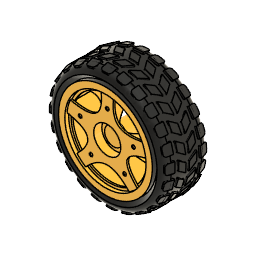
Rubber wheel (Autodesk Fusion 360 design; units mm, degrees)
part number: 2025-09-30-12-13-26-150
Autodesk Fusion 360 part; units mm, degrees
sketch "Sketch3" plane through (0, 0, 0) normal (0, 1, 0) x (1, 0, 0)
  circle A0 centre (0, 0) radius 26
  circle A1 centre (0, 0) radius 22.5
  dimension "d5" = 52
  dimension "d6" = 45
  constraint coincident A0.centre A1.centre
  measures "d5" diameter of A0
  measures "d6" diameter of A1
extrude "Extrude2" add sketch "Sketch3" along normal blind 25 makes body 1
sketch "Sketch4" plane through (0, 0, 0) normal (0, 1, 0) x (1, 0, 0)
  circle A0 centre (0, 0) radius 22.39
  dimension "d9" = 44.78
  constraint coincident A0.centre origin
  measures "d9" diameter of A0
extrude "Extrude3" add sketch "Sketch4" along normal blind 25 separate body makes body 2
sketch "Sketch5" plane through (0, 25, 0) normal (0, 1, 0) x (-1, 0, 0)
  circle A0 centre (0, 0) radius 22.39
  circle A1 centre (0, 0) radius 21
  dimension "d12" = 42
  constraint concentric A0 A1
  measures "d12" diameter of A1
extrude "Extrude4" cut sketch "Sketch5" against normal blind 20 contours A1 bodies 2
sketch "Sketch6" plane through (0, 0, 0) normal (0, 1, 0) x (1, 0, 0)
  circle A0 centre (0, 0) radius 21
  dimension "d15" = 42
  constraint coincident A0.centre origin
  measures "d15" diameter of A0
extrude "Extrude5" cut sketch "Sketch6" along normal blind 4 bodies 2
extrude "Extrude6" cut 1 faces at (-5.9246, 4, -2.0633) along direction (0, 1, 0) blind 1 on bodies 2 bodies 2
extrude "Extrude7" cut 1 faces at (21.7651, 25, 2.1556) along direction (0, -1, 0) blind 20 on bodies 2 bodies 2
extrude "Extrude8" cut 1 faces at (21.8433, 0, 1.1124) along direction (0, 1, 0) blind 4 on bodies 2 bodies 2
sketch "Sketch7" plane through (0, 0, 0) normal (0, 1, 0) x (1, 0, 0)
  circle A0 centre (0, 0) radius 9
  dimension "d24" = 18
  constraint coincident A0.centre origin
  measures "d24" diameter of A0
extrude "Extrude9" add sketch "Sketch7" along normal blind 25 separate body makes body 3
sketch "Sketch8" plane through (0, 0, 0) normal (0, 1, 0) x (1, 0, 0)
  circle A0 centre (0, 0) radius 7.5
  dimension "d27" = 15
  constraint coincident A0.centre origin
  measures "d27" diameter of A0
extrude "Extrude10" cut sketch "Sketch8" along normal blind 4 bodies 3
sketch "Sketch9" plane through (0, 25, 0) normal (0, 1, 0) x (-1, 0, 0)
  circle A0 centre (0, 0) radius 9
  circle A1 centre (0, 0) radius 5
  dimension "d30" = 10
  constraint coincident A0.centre A1.centre
  measures "d30" diameter of A1
extrude "Extrude11" cut sketch "Sketch9" against normal blind 20 bodies 3
sketch "Sketch10" plane through (0, 25, 0) normal (0, 1, 0) x (-1, 0, 0)
  circle A0 centre (0, 0) radius 5
  circle A1 centre (0, 0) radius 3
  dimension "d33" = 6
  constraint coincident A0.centre A1.centre
  measures "d33" diameter of A1
extrude "Extrude12" cut sketch "Sketch10" against normal blind 20 contours A1 bodies 3
sketch "Sketch11" plane through (0, 0, 0) normal (0, 1, 0) x (1, 0, 0)
  circle A0 centre (0, 0) radius 5
  dimension "d36" = 10
  constraint coincident A0.centre origin
  measures "d36" diameter of A0
extrude "Extrude13" add sketch "Sketch11" along normal blind 4 bodies 3
extrude "Extrude14" cut 1 faces at (1.3101, 0, 1.9935) along direction (0, 1, 0) blind 3 on bodies 3 bodies 3
sketch "Sketch12" plane through (0, 0, 0) normal (0, 1, 0) x (1, 0, 0)
  circle A0 centre (-4, -5) radius 0.5
  circle A1 centre (4, -5) radius 0.5
  circle A2 centre (-4, 5) radius 0.5
  circle A3 centre (4, 5) radius 0.5
  dimension "d41" = 1
  dimension "d42" = 1
  dimension "d43" = 1
  dimension "d44" = 1
  measures "d41" diameter of A0
  measures "d42" diameter of A1
  measures "d43" diameter of A2
  measures "d44" diameter of A3
extrude "Extrude15" add sketch "Sketch12" along normal blind 4 bodies 3
extrude "Extrude16" cut 4 faces at (-3.8778, 0, 5.1472) (4.1222, 0, 4.8866) (4.1222, 0, -5.1134) (-3.8778, 0, -4.8528) along direction (0, 1, 0) blind 3.5 on bodies 3 bodies 3
extrude "Extrude17" cut 1 faces at (1.3101, 3, 1.9935) along direction (0, 1, 0) blind 0.5 on bodies 3 bodies 3
extrude "Extrude18" cut 1 faces at (-2.7054, 4, 5.6176) along direction (0, 1, 0) blind 0.5 on bodies 3 bodies 3
extrude "Extrude19" cut 1 faces at (4.1222, 3.5, 4.8866) along direction (0, 1, 0) blind 0.5 on bodies 3 bodies 3
extrude "Extrude20" cut 3 faces at (-3.8778, 3.5, 5.1472) (-3.8778, 3.5, -4.8528) (4.1222, 3.5, -5.1134) along direction (0, 1, 0) blind 0.5 on bodies 3 bodies 3
extrude "Extrude21" cut 1 faces at (8.4386, 0, 0.8197) along direction (0, 1, 0) blind 0.5 on bodies 3 bodies 3
extrude "Extrude22" add 1 faces at (21.8433, 4, 1.1124) along direction (0, -1, 0) blind 0.5 on bodies 2 bodies 2
extrude "Extrude23" add 1 faces at (21.8433, 3.5, 1.1124) along direction (0, -1, 0) blind 1.5 on bodies 2 bodies 2
extrude "Extrude24" add 1 faces at (7.6145, 5, 0.6955) along direction (0, 1, 0) blind 1 on bodies 3 bodies 3
extrude "Extrude25" cut 1 faces at (1.3101, 3.5, 1.9935) along direction (0, 1, 0) blind 0.5 on bodies 3 bodies 3
extrude "Extrude26" cut 1 faces at (-2.7054, 4.5, 5.6176) along direction (0, 1, 0) blind 0.5 on bodies 3 bodies 3
extrude "Extrude27" cut 4 faces at (4.1222, 4, 4.8866) (-3.8778, 4, 5.1472) (-3.8778, 4, -4.8528) (4.1222, 4, -5.1134) along direction (0, 1, 0) blind 0.5 on bodies 3 bodies 3
extrude "Extrude28" cut 1 faces at (8.4386, 0.5, 0.8197) along direction (0, 1, 0) blind 0.5 on bodies 3 bodies 3
extrude "Extrude29" cut 1 faces at (1.3101, 4, 1.9935) along direction (0, 1, 0) blind 0.5 on bodies 3 bodies 3
extrude "Extrude30" cut 1 faces at (-2.7054, 5, 5.6176) along direction (0, 1, 0) blind 0.5 on bodies 3 bodies 3
extrude "Extrude31" cut 4 faces at (4.1222, 4.5, 4.8866) (-3.8778, 4.5, 5.1472) (-3.8778, 4.5, -4.8528) (4.1222, 4.5, -5.1134) along direction (0, 1, 0) blind 0.5 on bodies 3 bodies 3
extrude "Extrude32" cut 1 faces at (8.4386, 1, 0.8197) along direction (0, 1, 0) blind 0.5 on bodies 3 bodies 3
extrude "Extrude33" cut 1 faces at (21.7651, 5, 2.1556) along direction (0, -1, 0) blind 2 on bodies 2 bodies 2
sketch "Sketch14" plane through (0, 2, 0) normal (0, -1, 0) x (1, 0, 0)
  circle A0 centre (0, 0) radius 21
  circle A1 centre (0, 0) radius 22.39
  spline S0 degree 5 poles (-3.4973, 22.1152) (-3.4006, 21.4068) (-3.2459, 20.0296) (-3.1304, 18.0828) (-3.213, 15.729) (-3.7369, 13.2166) (-4.7167, 11.17) (-6.186, 9.6237) (-8.1564, 8.5893) (-10.6008, 8.0394) (-13.4805, 7.9342) (-16.1022, 8.1751) (-18.2359, 8.5267) (-19.7314, 8.8358) (-20.4975, 9.0091) knots 0 0 0 0 0 0 0.1 0.2 0.3 0.4 0.5 0.6 0.7 0.8 0.9 1 1 1 1 1 1
  spline S1 degree 5 poles (3.5817, 22.1017) (3.4802, 21.3937) (3.3163, 20.0174) (3.1876, 18.0719) (3.2545, 15.7198) (3.7619, 13.2094) (4.7285, 11.1648) (6.1881, 9.6202) (8.1522, 8.5873) (10.5935, 8.0385) (13.4729, 7.934) (16.0965, 8.1752) (18.2326, 8.5268) (19.7303, 8.8359) (20.4975, 9.0091) knots 0 0 0 0 0 0 0.1 0.2 0.3 0.4 0.5 0.6 0.7 0.8 0.9 1 1 1 1 1 1
  spline S2 degree 5 poles (-22.2999, 2.0065) (-21.5457, 1.858) (-20.0933, 1.5448) (-18.0826, 1.0258) (-15.7431, 0.2342) (-13.4268, -0.9327) (-11.7736, -2.2931) (-10.839, -3.8632) (-10.6558, -5.6526) (-11.1973, -7.6534) (-12.41, -9.8502) (-13.8739, -11.7516) (-15.2319, -13.2536) (-16.2509, -14.2882) (-16.7889, -14.8137) knots 0 0 0 0 0 0 0.1 0.2 0.3 0.4 0.5 0.6 0.7 0.8 0.9 1 1 1 1 1 1
  spline S3 degree 5 poles (-11.9561, -18.9305) (-11.4797, -18.4067) (-10.5263, -17.4047) (-9.0948, -16.0384) (-7.1832, -14.4945) (-4.7882, -13.0593) (-2.3875, -12.1628) (0.0196, -11.8488) (2.4332, -12.1407) (4.8531, -13.0142) (7.2788, -14.4252) (9.2236, -15.9486) (10.6845, -17.2991) (11.6593, -18.2903) (12.147, -18.8086) knots 0 0 0 0 0 0 0.1 0.2 0.3 0.4 0.5 0.6 0.7 0.8 0.9 1 1 1 1 1 1
  spline S4 degree 5 poles (22.2946, 2.0646) (21.5424, 1.9146) (20.0936, 1.5981) (18.0874, 1.0738) (15.7518, 0.2739) (13.4367, -0.9054) (11.7808, -2.2803) (10.8389, -3.8673) (10.6436, -5.676) (11.168, -7.6984) (12.3591, -9.9187) (13.8022, -11.8404) (15.1427, -13.3585) (16.1494, -14.404) (16.6809, -14.9352) knots 0 0 0 0 0 0 0.1 0.2 0.3 0.4 0.5 0.6 0.7 0.8 0.9 1 1 1 1 1 1
  point P0 (-6, 10)
  point P1 (6, 10)
  point P2 (-11, -4)
  point P3 (0, -12)
  point P4 (11, -4)
  constraint coincident A1 S0.start
  constraint coincident A1 S0.end
  constraint coincident A1 S1.start
  constraint coincident A1 S1.end
  constraint coincident A1 S2.start
  constraint coincident A1 S2.end
  constraint coincident A1 S3.start
  constraint coincident A1 S3.end
  constraint coincident A1 S4.start
  constraint coincident A1 S4.end
extrude "Extrude34" add sketch "Sketch14" along normal blind 0.01 contours A0 S0 S1 S2 S3 S4 | A0 A1 S1 S4 | A0 A1 S3 S4 | A0 A1 S0 S1 | A0 A1 S2 S3 | A0 A1 S0 S2 bodies 2 3
extrude "Extrude35" add 1 faces at (8.4386, 1.5, 0.8197) along direction (0, -1, 0) blind 0.5 on bodies 2 bodies 2
extrude "Extrude36" add 1 faces at (-12.1299, 1.99, 3.4531) along direction (0, -1, 0) blind 0.95 on bodies 2 bodies 2
extrude "Extrude37" add 1 faces at (-12.1299, 1.04, 3.4531) along direction (0, -1, 0) blind 0.04 on bodies 2 bodies 2
extrude "Extrude38" cut 1 faces at (1.9158, 1.99, 2.8099) along direction (0, 1, 0) blind 2 on bodies 2 bodies 2
fillet "Fillet1" radius 3 1 edges at (-8.3909, 6, 3.2545) on bodies 2
sketch "Sketch15" plane through (0, 2, 0) normal (0, 1, 0) x (-1, 0, 0)
  circle A0 centre (0, 0) radius 9
  arc A1 (-19.1063, 8.7148) -> (-20.9251, 1.7721) centre (0, 0) ccw
  spline S0 degree 5 poles (-20.9251, 1.7721) (-20.4807, 1.6705) (-19.3542, 1.3982) (-17.6543, 0.9227) (-15.5784, 0.1856) (-13.4367, -0.9054) (-11.7808, -2.2803) (-10.8389, -3.8673) (-10.6436, -5.676) (-11.168, -7.6984) (-12.2684, -9.7495) (-13.5318, -11.4758) (-14.6447, -12.784) (-15.4072, -13.6149) (-15.7096, -13.9358) knots 0.037451 0.037451 0.037451 0.037451 0.037451 0.037451 0.1 0.2 0.3 0.4 0.5 0.6 0.7 0.8 0.9 0.961913 0.961913 0.961913 0.961913 0.961913 0.961913
  arc A2 (-15.7096, -13.9358) -> (-11.1555, -17.792) centre (0, 0) ccw
  spline S1 degree 5 poles (10.9829, -17.899) (10.7008, -17.6112) (9.9416, -16.8584) (8.7045, -15.7273) (6.9876, -14.3773) (4.7882, -13.0593) (2.3875, -12.1628) (-0.0196, -11.8488) (-2.4332, -12.1407) (-4.8531, -13.0142) (-7.0814, -14.3104) (-8.8281, -15.6429) (-10.0903, -16.7612) (-10.8664, -17.5065) (-11.1555, -17.792) knots 0.040836 0.040836 0.040836 0.040836 0.040836 0.040836 0.1 0.2 0.3 0.4 0.5 0.6 0.7 0.8 0.9 0.959321 0.959321 0.959321 0.959321 0.959321 0.959321
  arc A3 (10.9829, -17.899) -> (15.8065, -13.8258) centre (0, 0) ccw
  spline S2 degree 5 poles (20.9296, 1.7176) (20.4835, 1.617) (19.3537, 1.3473) (17.6496, 0.8766) (15.57, 0.147) (13.4268, -0.9327) (11.7736, -2.2931) (10.839, -3.8632) (10.6558, -5.6526) (11.1973, -7.6534) (12.3177, -9.683) (13.5998, -11.3912) (14.7277, -12.6858) (15.5001, -13.5081) (15.8065, -13.8258) knots 0.037374 0.037374 0.037374 0.037374 0.037374 0.037374 0.1 0.2 0.3 0.4 0.5 0.6 0.7 0.8 0.9 0.961948 0.961948 0.961948 0.961948 0.961948 0.961948
  arc A4 (20.9296, 1.7176) -> (19.1065, 8.7144) centre (0, 0) ccw
  spline S3 degree 5 poles (3.3353, 20.7335) (3.2958, 20.3268) (3.2093, 19.2625) (3.1502, 17.6167) (3.2548, 15.5285) (3.7369, 13.2166) (4.7167, 11.17) (6.186, 9.6237) (8.1564, 8.5893) (10.6008, 8.0394) (13.2675, 7.942) (15.6203, 8.1333) (17.4548, 8.4045) (18.6407, 8.6226) (19.1065, 8.7144) knots 0.039901 0.039901 0.039901 0.039901 0.039901 0.039901 0.1 0.2 0.3 0.4 0.5 0.6 0.7 0.8 0.9 0.963032 0.963032 0.963032 0.963032 0.963032 0.963032
  arc A5 (3.3353, 20.7335) -> (-3.4104, 20.7212) centre (0, 0) ccw
  spline S4 degree 5 poles (-3.4104, 20.7212) (-3.3681, 20.3147) (-3.2745, 19.251) (-3.2043, 17.6062) (-3.295, 15.5195) (-3.7619, 13.2094) (-4.7285, 11.1648) (-6.1881, 9.6202) (-8.1522, 8.5873) (-10.5935, 8.0385) (-13.2603, 7.9418) (-15.6149, 8.1334) (-17.4516, 8.4048) (-18.6395, 8.623) (-19.1063, 8.7148) knots 0.039888 0.039888 0.039888 0.039888 0.039888 0.039888 0.1 0.2 0.3 0.4 0.5 0.6 0.7 0.8 0.9 0.963081 0.963081 0.963081 0.963081 0.963081 0.963081
  line L0 (0.4907, 5.8974) -> (-0.5093, 5.8974)
  line L1 (-0.5093, 5.8974) -> (-0.5093, 22.3974)
  line L2 (-0.5093, 22.3974) -> (0.4907, 22.3974)
  line L3 (0.4907, 22.3974) -> (0.4907, 5.8974)
  line L4 (0.4907, 5.8974) -> (-0.5093, 22.3974) construction
  line L5 (-0.5093, 5.8974) -> (0.4907, 22.3974) construction
  point P0 (-0.0093, 14.1474)
  dimension "d97" = 16.5
  dimension "d104" = 1
  constraint horizontal L0
  constraint perpendicular L0 L1
  constraint parallel L0 L2
  constraint parallel L1 L3
  constraint coincident L4 P0
  constraint coincident L5 P0
  measures "d97" distance of L0.start L2.end
  measures "d104" distance of L0.start L0.end
extrude "Extrude39" add sketch "Sketch15" along normal blind 50 separate body contours A0 L0 L1 L3 | A0 A5 L1 L3 | A5 L1 L2 L3 picked at (-0.0649, 6.931) makes body 4
move_body "Move1" bodies 4 to x (1, 0, 0) y (0, 1, 0) z (0, 0, 1) at (0, 25, 0)
sketch "Sketch16" plane through (0.5093, 0, 0) normal (1, 0, 0) x (0, 1, 0)
  line L0 (27, 22.3974) -> (27, 5.8974)
  line L1 (27, 5.8974) -> (77, 5.8974)
  line L2 (77, 5.8974) -> (77, 22.3974)
  line L3 (77, 22.3974) -> (27, 22.3974)
  spline S0 degree 5 poles (38.1111, 22.3974) (38.1988, 22.195) (38.3552, 21.7856) (38.5326, 21.1581) (38.6539, 20.2941) (38.6109, 19.1683) (38.3743, 17.9982) (37.9532, 16.7885) (37.371, 15.5487) (36.6689, 14.295) (35.8984, 13.0469) (35.1155, 11.8254) (34.3741, 10.6507) (33.7208, 9.54) (33.1872, 8.5045) (32.7879, 7.5487) (32.5801, 6.8485) (32.4868, 6.3591) (32.4521, 6.0487) (32.4417, 5.8974) knots 0 0 0 0 0 0 0.066667 0.133333 0.2 0.266667 0.333333 0.4 0.466667 0.533333 0.6 0.666667 0.733333 0.8 0.866667 0.933333 1 1 1 1 1 1
  point P0 (38, 17)
  point P1 (34, 10)
  constraint coincident L3 S0.start
  constraint coincident L1 S0.end
extrude "Extrude40" cut sketch "Sketch16" against normal blind 4 contours L1 L2 L3 S0 bodies 4
move_body "Move2" bodies 4 to x (1, 0, 0) y (0, 1, 0) z (0, 0, 1) at (0, 15, 0)
sketch "Sketch17" plane through (0.5093, 0, 0) normal (1, 0, 0) x (0, 1, 0)
  line L0 (53.1111, 22.3974) -> (42, 22.3974)
  line L1 (42, 22.3974) -> (42, 5.8974)
  line L2 (42, 5.8974) -> (47.4417, 5.8974)
  spline S0 degree 5 poles (42, 9) (42.1601, 9.0078) (42.4742, 9.0173) (42.9273, 9.0136) (43.4948, 8.9722) (44.1387, 8.8552) (44.7112, 8.667) (45.2057, 8.401) (45.6178, 8.053) (45.9494, 7.6247) (46.206, 7.1217) (46.3559, 6.6642) (46.4391, 6.2919) (46.4818, 6.031) (46.5, 5.8974) knots 0 0 0 0 0 0 0.1 0.2 0.3 0.4 0.5 0.6 0.7 0.8 0.9 1 1 1 1 1 1
  spline S1 degree 5 poles (47.4417, 5.8974) (47.4521, 6.0487) (47.4868, 6.3591) (47.5801, 6.8485) (47.7879, 7.5487) (48.1872, 8.5045) (48.7208, 9.54) (49.3741, 10.6507) (50.1155, 11.8254) (50.8984, 13.0469) (51.6689, 14.295) (52.371, 15.5487) (52.9532, 16.7885) (53.3743, 17.9982) (53.6109, 19.1683) (53.6539, 20.2941) (53.5326, 21.1581) (53.3552, 21.7856) (53.1988, 22.195) (53.1111, 22.3974) knots -1 -1 -1 -1 -1 -1 -0.933333 -0.866667 -0.8 -0.733333 -0.666667 -0.6 -0.533333 -0.466667 -0.4 -0.333333 -0.266667 -0.2 -0.133333 -0.066667 0 0 0 0 0 0
  point P0 (45.2689, 8.3214)
  constraint coincident L1 S0.start
  constraint coincident L2 S0.end
extrude "Extrude41" cut sketch "Sketch17" against normal blind 4 contours L1 L2 S0 bodies 4
move_body "Move3" bodies 4 to x (1, 0, 0) y (0, 1, 0) z (0, 0, 1) at (0, -40, 0)
copy_body "CopyPasteBodies1" bodies 4 makes body 5
move_body "Move4" bodies 5 to x (0.258819, 0, 0.965926) y (0, 1, 0) z (-0.965926, 0, 0.258819) at (0.0096, 0, 0.3239)
copy_body "CopyPasteBodies2" bodies 4 makes body 6
move_body "Move5" bodies 6 to x (0.207912, 0, -0.978148) y (0, 1, 0) z (0.978148, 0, 0.207912) at (-0.2765, 0, 1.1348)
copy_body "CopyPasteBodies3" bodies 6 makes body 7
move_body "Move6" bodies 7 to x (0.5, 0, -0.866025) y (0, 1, 0) z (0.866025, 0, 0.5) at (-1.3001, 0, -1.3816)
copy_body "CopyPasteBodies4" bodies 4 makes body 8
move_body "Move7" bodies 8 to x (-0.766044, 0, 0.642788) y (0, 1, 0) z (-0.642788, 0, -0.766044) at (-0.0954, -3, -0.0152)
move_body "Move8" bodies 8 to x (1, 0, 0) y (0, 1, 0) z (0, 0, 1) at (0, 3, 0)
sketch "Sketch18" plane through (0, 0, 0) normal (0, 1, 0) x (1, 0, 0)
  circle A0 centre (0, 0) radius 32.5
  circle A1 centre (0, 0) radius 26
  dimension "d106" = 65
  dimension "d107" = 52
  constraint coincident A0.centre A1.centre
  measures "d106" diameter of A0
  measures "d107" diameter of A1
extrude "Extrude42" add sketch "Sketch18" along normal blind 25 separate body makes body 9
chamfer "Chamfer2" distance 2.6 angle 45 1 edges at (-24.2405, 0, -9.402) on bodies 9
chamfer "Chamfer3" distance 2.6 angle 45 1 edges at (-24.2405, 25, -9.402) on bodies 9
fillet "Fillet2" radius 4 2 edges at (-30.3006, 0, 11.7525) (-30.3006, 25, 11.7525) on bodies 9
ref_plane "WorkPlane1" through (0, 0, 32.5) normal (0, 0, 1) x (1, 0, 0)
sketch "Sketch21" plane through (0, 0, 32.5) normal (0, 0, 1) x (1, 0, 0)
  line L0 (0.1437, 20.1039) -> (5.1437, 20.1039)
  line L1 (3, 16) -> (8, 16)
  line L2 (0.1437, 20.1039) -> (3, 16)
  line L3 (5.1437, 20.1039) -> (8, 16)
  line L4 (-0.3871, 10.4839) -> (4.6129, 10.4839)
  line L5 (-3.3871, 6.4839) -> (1.6129, 6.4839)
  line L6 (-0.3871, 10.4839) -> (-3.3871, 6.4839)
  line L7 (4.6129, 10.4839) -> (1.6129, 6.4839)
  dimension "d130" = 5
  dimension "d131" = 5
  dimension "d132" = 5
  dimension "d133" = 5
  dimension "d134" = 5
  dimension "d135" = 5
  constraint horizontal L0
  constraint parallel L0 L1
  constraint horizontal L4
  constraint parallel L4 L5
  measures "d130" distance of L0.start L0.end
  measures "d131" distance of L1.start L1.end
  measures "d132" distance of L0.start L1.start
  measures "d133" distance of L4.start L4.end
  measures "d134" distance of L5.start L5.end
  measures "d135" distance of L4.start L5.start
sketch "Sketch23" plane through (0, 1, 0) normal (0, -1, 0) x (1, 0, 0)
  arc A0 (3.5817, 22.1017) -> (-3.4973, 22.1152) centre (0, 0) ccw
  spline S0 degree 5 poles (-3.4973, 22.1152) (-3.4006, 21.4068) (-3.2459, 20.0296) (-3.1304, 18.0828) (-3.213, 15.729) (-3.7369, 13.2166) (-4.7167, 11.17) (-6.186, 9.6237) (-8.1564, 8.5893) (-10.6008, 8.0394) (-13.4805, 7.9342) (-16.1022, 8.1751) (-18.2359, 8.5267) (-19.7314, 8.8358) (-20.4975, 9.0091) knots 0 0 0 0 0 0 0.1 0.2 0.3 0.4 0.5 0.6 0.7 0.8 0.9 1 1 1 1 1 1
  arc A1 (-20.4975, 9.0091) -> (-22.2999, 2.0065) centre (0, 0) ccw
  spline S1 degree 5 poles (-22.2999, 2.0065) (-21.5457, 1.858) (-20.0933, 1.5448) (-18.0826, 1.0258) (-15.7431, 0.2342) (-13.4268, -0.9327) (-11.7736, -2.2931) (-10.839, -3.8632) (-10.6558, -5.6526) (-11.1973, -7.6534) (-12.41, -9.8502) (-13.8739, -11.7516) (-15.2319, -13.2536) (-16.2509, -14.2882) (-16.7889, -14.8137) knots 0 0 0 0 0 0 0.1 0.2 0.3 0.4 0.5 0.6 0.7 0.8 0.9 1 1 1 1 1 1
  arc A2 (-16.7889, -14.8137) -> (-11.9561, -18.9305) centre (0, 0) ccw
  spline S2 degree 5 poles (-11.9561, -18.9305) (-11.4797, -18.4067) (-10.5263, -17.4047) (-9.0948, -16.0384) (-7.1832, -14.4945) (-4.7882, -13.0593) (-2.3875, -12.1628) (0.0196, -11.8488) (2.4332, -12.1407) (4.8531, -13.0142) (7.2788, -14.4252) (9.2236, -15.9486) (10.6845, -17.2991) (11.6593, -18.2903) (12.147, -18.8086) knots 0 0 0 0 0 0 0.1 0.2 0.3 0.4 0.5 0.6 0.7 0.8 0.9 1 1 1 1 1 1
  arc A3 (12.147, -18.8086) -> (16.6809, -14.9352) centre (0, 0) ccw
  spline S3 degree 5 poles (16.6809, -14.9352) (16.1494, -14.404) (15.1427, -13.3585) (13.8022, -11.8404) (12.3591, -9.9187) (11.168, -7.6984) (10.6436, -5.676) (10.8389, -3.8673) (11.7808, -2.2803) (13.4367, -0.9054) (15.7518, 0.2739) (18.0874, 1.0738) (20.0936, 1.5981) (21.5424, 1.9146) (22.2946, 2.0646) knots -1 -1 -1 -1 -1 -1 -0.9 -0.8 -0.7 -0.6 -0.5 -0.4 -0.3 -0.2 -0.1 0 0 0 0 0 0
  arc A4 (22.2946, 2.0646) -> (20.4975, 9.0091) centre (0, 0) ccw
  spline S4 degree 5 poles (20.4975, 9.0091) (19.7303, 8.8359) (18.2326, 8.5268) (16.0965, 8.1752) (13.4729, 7.934) (10.5935, 8.0385) (8.1522, 8.5873) (6.1881, 9.6202) (4.7285, 11.1648) (3.7619, 13.2094) (3.2545, 15.7198) (3.1876, 18.0719) (3.3163, 20.0174) (3.4802, 21.3937) (3.5817, 22.1017) knots -1 -1 -1 -1 -1 -1 -0.9 -0.8 -0.7 -0.6 -0.5 -0.4 -0.3 -0.2 -0.1 0 0 0 0 0 0
  circle A5 centre (0, 0) radius 7.5
  circle A6 centre (14.4935, 3.8649) radius 1
  dimension "d138" = 2
  dimension "d139" = 15
  measures "d138" diameter of A6
  measures "d139" distance of A0.centre A6.centre
extrude "Extrude48" cut sketch "Sketch23" against normal blind 0.5 contours A6 bodies 2
sketch "Sketch24" plane through (0, 1, 0) normal (0, -1, 0) x (1, 0, 0)
  circle A0 centre (14.4935, 3.8649) radius 1
  arc A1 (3.5817, 22.1017) -> (-3.4973, 22.1152) centre (0, 0) ccw
  spline S0 degree 5 poles (-3.4973, 22.1152) (-3.4006, 21.4068) (-3.2459, 20.0296) (-3.1304, 18.0828) (-3.213, 15.729) (-3.7369, 13.2166) (-4.7167, 11.17) (-6.186, 9.6237) (-8.1564, 8.5893) (-10.6008, 8.0394) (-13.4805, 7.9342) (-16.1022, 8.1751) (-18.2359, 8.5267) (-19.7314, 8.8358) (-20.4975, 9.0091) knots 0 0 0 0 0 0 0.1 0.2 0.3 0.4 0.5 0.6 0.7 0.8 0.9 1 1 1 1 1 1
  arc A2 (-20.4975, 9.0091) -> (-22.2999, 2.0065) centre (0, 0) ccw
  spline S1 degree 5 poles (-22.2999, 2.0065) (-21.5457, 1.858) (-20.0933, 1.5448) (-18.0826, 1.0258) (-15.7431, 0.2342) (-13.4268, -0.9327) (-11.7736, -2.2931) (-10.839, -3.8632) (-10.6558, -5.6526) (-11.1973, -7.6534) (-12.41, -9.8502) (-13.8739, -11.7516) (-15.2319, -13.2536) (-16.2509, -14.2882) (-16.7889, -14.8137) knots 0 0 0 0 0 0 0.1 0.2 0.3 0.4 0.5 0.6 0.7 0.8 0.9 1 1 1 1 1 1
  arc A3 (-16.7889, -14.8137) -> (-11.9561, -18.9305) centre (0, 0) ccw
  spline S2 degree 5 poles (-11.9561, -18.9305) (-11.4797, -18.4067) (-10.5263, -17.4047) (-9.0948, -16.0384) (-7.1832, -14.4945) (-4.7882, -13.0593) (-2.3875, -12.1628) (0.0196, -11.8488) (2.4332, -12.1407) (4.8531, -13.0142) (7.2788, -14.4252) (9.2236, -15.9486) (10.6845, -17.2991) (11.6593, -18.2903) (12.147, -18.8086) knots 0 0 0 0 0 0 0.1 0.2 0.3 0.4 0.5 0.6 0.7 0.8 0.9 1 1 1 1 1 1
  arc A4 (12.147, -18.8086) -> (16.6809, -14.9352) centre (0, 0) ccw
  spline S3 degree 5 poles (16.6809, -14.9352) (16.1494, -14.404) (15.1427, -13.3585) (13.8022, -11.8404) (12.3591, -9.9187) (11.168, -7.6984) (10.6436, -5.676) (10.8389, -3.8673) (11.7808, -2.2803) (13.4367, -0.9054) (15.7518, 0.2739) (18.0874, 1.0738) (20.0936, 1.5981) (21.5424, 1.9146) (22.2946, 2.0646) knots -1 -1 -1 -1 -1 -1 -0.9 -0.8 -0.7 -0.6 -0.5 -0.4 -0.3 -0.2 -0.1 0 0 0 0 0 0
  arc A5 (22.2946, 2.0646) -> (20.4975, 9.0091) centre (0, 0) ccw
  spline S4 degree 5 poles (20.4975, 9.0091) (19.7303, 8.8359) (18.2326, 8.5268) (16.0965, 8.1752) (13.4729, 7.934) (10.5935, 8.0385) (8.1522, 8.5873) (6.1881, 9.6202) (4.7285, 11.1648) (3.7619, 13.2094) (3.2545, 15.7198) (3.1876, 18.0719) (3.3163, 20.0174) (3.4802, 21.3937) (3.5817, 22.1017) knots -1 -1 -1 -1 -1 -1 -0.9 -0.8 -0.7 -0.6 -0.5 -0.4 -0.3 -0.2 -0.1 0 0 0 0 0 0
  circle A6 centre (0, 0) radius 7.5
  circle A7 centre (0, 15) radius 1
  circle A8 centre (-15, 4) radius 1
  circle A9 centre (-9, -11.5) radius 1
  circle A10 centre (9.4986, -11.6094) radius 1
  dimension "d142" = 2
  dimension "d143" = 15
  dimension "d144" = 2
  dimension "d145" = 15
  dimension "d146" = 2
  dimension "d147" = 11.5
  dimension "d148" = 2
  dimension "d149" = 15
  measures "d142" diameter of A7
  measures "d143" distance of A1.centre A7.centre
  measures "d144" diameter of A8
  measures "d145" horizontal distance of A1.centre A8.centre
  measures "d146" diameter of A9
  measures "d147" vertical distance of A1.centre A9.centre
  measures "d148" diameter of A10
  measures "d149" distance of A1.centre A10.centre
extrude "Extrude49" cut sketch "Sketch24" against normal blind 0.5 contours A7 | A8 | A9 bodies 2
sketch "Sketch25" plane through (0, 1, 0) normal (0, -1, 0) x (1, 0, 0)
  circle A0 centre (0, 15) radius 1
  circle A1 centre (-15, 4) radius 1
  circle A2 centre (-9, -11.5) radius 1
  circle A3 centre (14.4935, 3.8649) radius 1
  arc A4 (3.5817, 22.1017) -> (-3.4973, 22.1152) centre (0, 0) ccw
  spline S0 degree 5 poles (-3.4973, 22.1152) (-3.4006, 21.4068) (-3.2459, 20.0296) (-3.1304, 18.0828) (-3.213, 15.729) (-3.7369, 13.2166) (-4.7167, 11.17) (-6.186, 9.6237) (-8.1564, 8.5893) (-10.6008, 8.0394) (-13.4805, 7.9342) (-16.1022, 8.1751) (-18.2359, 8.5267) (-19.7314, 8.8358) (-20.4975, 9.0091) knots 0 0 0 0 0 0 0.1 0.2 0.3 0.4 0.5 0.6 0.7 0.8 0.9 1 1 1 1 1 1
  arc A5 (-20.4975, 9.0091) -> (-22.2999, 2.0065) centre (0, 0) ccw
  spline S1 degree 5 poles (-22.2999, 2.0065) (-21.5457, 1.858) (-20.0933, 1.5448) (-18.0826, 1.0258) (-15.7431, 0.2342) (-13.4268, -0.9327) (-11.7736, -2.2931) (-10.839, -3.8632) (-10.6558, -5.6526) (-11.1973, -7.6534) (-12.41, -9.8502) (-13.8739, -11.7516) (-15.2319, -13.2536) (-16.2509, -14.2882) (-16.7889, -14.8137) knots 0 0 0 0 0 0 0.1 0.2 0.3 0.4 0.5 0.6 0.7 0.8 0.9 1 1 1 1 1 1
  arc A6 (-16.7889, -14.8137) -> (-11.9561, -18.9305) centre (0, 0) ccw
  spline S2 degree 5 poles (-11.9561, -18.9305) (-11.4797, -18.4067) (-10.5263, -17.4047) (-9.0948, -16.0384) (-7.1832, -14.4945) (-4.7882, -13.0593) (-2.3875, -12.1628) (0.0196, -11.8488) (2.4332, -12.1407) (4.8531, -13.0142) (7.2788, -14.4252) (9.2236, -15.9486) (10.6845, -17.2991) (11.6593, -18.2903) (12.147, -18.8086) knots 0 0 0 0 0 0 0.1 0.2 0.3 0.4 0.5 0.6 0.7 0.8 0.9 1 1 1 1 1 1
  arc A7 (12.147, -18.8086) -> (16.6809, -14.9352) centre (0, 0) ccw
  spline S3 degree 5 poles (16.6809, -14.9352) (16.1494, -14.404) (15.1427, -13.3585) (13.8022, -11.8404) (12.3591, -9.9187) (11.168, -7.6984) (10.6436, -5.676) (10.8389, -3.8673) (11.7808, -2.2803) (13.4367, -0.9054) (15.7518, 0.2739) (18.0874, 1.0738) (20.0936, 1.5981) (21.5424, 1.9146) (22.2946, 2.0646) knots -1 -1 -1 -1 -1 -1 -0.9 -0.8 -0.7 -0.6 -0.5 -0.4 -0.3 -0.2 -0.1 0 0 0 0 0 0
  arc A8 (22.2946, 2.0646) -> (20.4975, 9.0091) centre (0, 0) ccw
  spline S4 degree 5 poles (20.4975, 9.0091) (19.7303, 8.8359) (18.2326, 8.5268) (16.0965, 8.1752) (13.4729, 7.934) (10.5935, 8.0385) (8.1522, 8.5873) (6.1881, 9.6202) (4.7285, 11.1648) (3.7619, 13.2094) (3.2545, 15.7198) (3.1876, 18.0719) (3.3163, 20.0174) (3.4802, 21.3937) (3.5817, 22.1017) knots -1 -1 -1 -1 -1 -1 -0.9 -0.8 -0.7 -0.6 -0.5 -0.4 -0.3 -0.2 -0.1 0 0 0 0 0 0
  circle A9 centre (0, 0) radius 7.5
  circle A10 centre (9.598, -11.5273) radius 1
  dimension "d152" = 2
  dimension "d153" = 15
  measures "d152" diameter of A10
  measures "d153" distance of A4.centre A10.centre
extrude "Extrude50" cut sketch "Sketch25" against normal blind 0.5 contours A10 bodies 2
ref_plane "WorkPlane2" through (0, 0, 32.5) normal (0, 0, 1) x (1, 0, 0)
sketch "Sketch26" plane through (0, 0, 32.5) normal (0, 0, 1) x (1, 0, 0)
  line L0 (2, 10) -> (7, 10)
  line L1 (-0.8618, 5.9) -> (4.1382, 5.9)
  line L2 (2, 10) -> (-0.8618, 5.9)
  line L3 (7, 10) -> (4.1382, 5.9)
  dimension "d157" = 5
  dimension "d158" = 5
  dimension "d159" = 4.1
  constraint horizontal L0
  constraint parallel L0 L1
  constraint parallel L2 L3
  measures "d157" distance of L0.start L0.end
  measures "d158" distance of L0.end L1.end
  measures "d159" distance of L0 L1
extrude "Extrude51" add sketch "Sketch26" along normal blind 1 separate body makes body 10
move_body "Move9" bodies 10 to x (0.99263, 0.002488, -0.121163) y (-0.005108, 0.99976, -0.021311) z (0.121081, 0.021773, 0.992404) at (-3.9443, -0.7359, 0.5968)
move_body "Move10" bodies 10 to x (0.996314, -0.000663, 0.08578) y (-0.000663, 0.999881, 0.015425) z (-0.08578, -0.015425, 0.996195) at (0.4137, 0.0744, -0.4555)
move_body "Move11" bodies 10 to x (1, 0, 0) y (0, 1, 0) z (0, 0, 1) at (-0.0078, 1.9999, -0.0125)
copy_body "CopyPasteBodies5" bodies 10 makes body 11
move_body "Move12" bodies 11 to x (-0.571594, 0.818976, 0.050584) y (-0.818263, -0.573512, 0.039109) z (0.06104, -0.019037, 0.997954) at (6.9149, 21.0581, -0.3801)
ref_plane "WorkPlane3" through (0, 0, 32.5) normal (0, 0, 1) x (1, 0, 0)
sketch "Sketch27" plane through (0, 0, 32.5) normal (0, 0, 1) x (1, 0, 0)
  line L0 (2.5, 2.3333) -> (-3, 2.3333)
  line L1 (-3, 2.3333) -> (-3, 6.8333)
  line L2 (-3, 6.8333) -> (2.5, 6.8333)
  line L3 (2.5, 6.8333) -> (2.5, 2.3333)
  line L4 (2.5, 2.3333) -> (-3, 6.8333) construction
  line L5 (-3, 2.3333) -> (2.5, 6.8333) construction
  point P0 (-0.25, 4.5833)
  dimension "d163" = 5.5
  dimension "d164" = 4.5
  constraint horizontal L0
  constraint perpendicular L0 L1
  constraint parallel L0 L2
  constraint parallel L1 L3
  constraint coincident L4 P0
  constraint coincident L5 P0
  measures "d163" distance of L1.end L2.end
  measures "d164" distance of L0.start L2.end
extrude "Extrude52" add sketch "Sketch27" along normal blind 1 separate body makes body 12
fillet "Fillet3" radius 1.5 2 edges at (-3, 2.3333, 33) (2.5, 2.3333, 33) on bodies 12
move_body "Move13" bodies 12 to x (1, 0, 0) y (0, 0.965926, 0.258819) z (0, -0.258819, 0.965926) at (-1, 7.3656, -0.9208)
copy_body "CopyPasteBodies6" bodies 12 makes body 13
move_body "Move14" bodies 13 to x (-0.996195, -0.007596, -0.086824) y (0.007596, -0.999971, 0.00033) z (-0.086824, -0.00033, 0.996224) at (0.1324, 24.9366, 0.0754)
pattern_circular "C-Pattern1" count 24 over 360 about axis through (0, 21.0013, 0) along (0, 1, 0) of bodies 11 10 12 13 makes body 14 at (7.6521, 8.8123, 31.2315) makes body 15 at (15.4747, 8.8123, 28.1868) makes body 16 at (22.2427, 8.8123, 23.2212) makes body 17 at (27.4949, 8.8123, 16.6732) makes body 18 at (30.8734, 8.8123, 8.9888) makes body 19 at (32.1479, 8.8123, 0.6919) makes body 20 at (31.2315, 8.8123, -7.6521) makes body 21 at (26.792, 10.1887, -17.6873) makes body 22 at (23.2212, 8.8123, -22.2427) makes body 23 at (16.6732, 8.8123, -27.4949) makes body 24 at (8.9888, 8.8123, -30.8734) makes body 25 at (0.6919, 8.8123, -32.1479) makes body 26 at (-7.6521, 8.8123, -31.2315) makes body 27 at (-15.4747, 8.8123, -28.1868) makes body 28 at (-24.0189, 10.1887, -21.3013) makes body 29 at (-27.4949, 8.8123, -16.6732) makes body 30 at (-31.8478, 8.8187, -9.2132) makes body 31 at (-32.1479, 8.8123, -0.6919) makes body 32 at (10.2769, 14.8255, 30.3872) makes body 33 at (17.7915, 14.8255, 26.6919) makes body 34 at (24.0937, 14.8255, 21.1776) makes body 35 at (28.3972, 16.1849, 17.0058) makes body 36 at (31.4545, 14.8255, 6.2936) makes body 37 at (32.0116, 14.8255, -2.0619) makes body 38 at (31.3433, 14.8319, -10.5698) makes body 39 at (26.6919, 14.8255, -17.7915) makes body 40 at (21.1776, 14.8255, -24.0937) makes body 41 at (17.0058, 16.1849, -28.3972) makes body 42 at (6.2936, 14.8255, -31.4545) makes body 43 at (-2.0619, 14.8255, -32.0116) makes body 44 at (-10.2769, 14.8255, -30.3872) makes body 45 at (-17.7915, 14.8255, -26.6919) makes body 46 at (-24.0937, 14.8255, -21.1776) makes body 47 at (-28.7539, 14.8255, -14.2201) makes body 48 at (-31.4545, 14.8255, -6.2936) makes body 49 at (-32.0116, 14.8255, 2.0619) makes body 50 at (6.1846, 4.5886, 31.4526) makes body 51 at (14.5974, 4.3297, 29.6167) makes body 52 at (21.0823, 4.5886, 24.1465) makes body 53 at (26.6135, 4.5886, 17.8672) makes body 54 at (30.3311, 4.5886, 10.3703) makes body 55 at (32.9475, 4.3297, 2.1667) makes body 56 at (31.4526, 4.5886, -6.1846) makes body 57 at (29.6167, 4.3297, -14.5974) makes body 58 at (24.1465, 4.5886, -21.0823) makes body 59 at (18.3501, 4.3297, -27.45) makes body 60 at (10.6203, 4.3297, -31.2641) makes body 61 at (2.1667, 4.5886, -31.9816) makes body 62 at (-6.1846, 4.5886, -31.4526) makes body 63 at (-14.5974, 4.3297, -29.6167) makes body 64 at (-21.7653, 4.3297, -24.8295) makes body 65 at (-26.6135, 4.5886, -17.8672) makes body 66 at (-30.3311, 4.5886, -10.3703) makes body 67 at (-32.9475, 4.3297, -2.1667) makes body 68 at (6.1877, 21.5646, 32.1652) makes body 69 at (14.3018, 21.5646, 29.4677) makes body 70 at (22.3975, 20.354, 23.0354) makes body 71 at (27.5963, 20.354, 16.4536) makes body 72 at (30.9145, 20.354, 8.7505) makes body 73 at (32.1259, 20.354, 0.4511) makes body 74 at (32.1652, 21.5646, -6.1877) makes body 75 at (27.8162, 21.32, -15.5563) makes body 76 at (23.0354, 20.354, -22.3975) makes body 77 at (16.8668, 21.5785, -28.1706) makes body 78 at (8.7505, 20.354, -30.9145) makes body 79 at (0.5369, 20.6125, -33.0881) makes body 80 at (-6.1877, 21.5646, -32.1652) makes body 81 at (-16.0791, 20.6125, -28.9236) makes body 82 at (-22.2256, 21.32, -22.8421) makes body 83 at (-27.3803, 21.32, -16.3114) makes body 84 at (-30.9145, 20.354, -8.7505) makes body 85 at (-32.1259, 20.354, -0.4511) makes body 86 at (-31.2315, 8.8123, 7.6521) makes body 87 at (-28.1868, 8.8123, 15.4747) makes body 88 at (-23.2212, 8.8123, 22.2427) makes body 89 at (-16.6732, 8.8123, 27.4949) makes body 90 at (-8.9888, 8.8123, 30.8734) makes body 91 at (-30.3872, 14.8255, 10.2769) makes body 92 at (-26.6919, 14.8255, 17.7915) makes body 93 at (-21.1776, 14.8255, 24.0937) makes body 94 at (-14.2201, 14.8255, 28.7539) makes body 95 at (-8.8523, 16.1785, 30.8566) makes body 96 at (-31.4526, 4.5886, 6.1846) makes body 97 at (-29.6167, 4.3297, 14.5974) makes body 98 at (-24.1465, 4.5886, 21.0823) makes body 99 at (-17.8672, 4.5886, 26.6135) makes body 100 at (-10.6203, 4.3297, 31.2641) makes body 101 at (-32.4185, 20.5986, 6.2399) makes body 102 at (-29.4677, 21.5646, 14.3018) makes body 103 at (-23.0354, 20.354, 22.3975) makes body 104 at (-16.3114, 21.32, 27.3803) makes body 105 at (-8.7505, 20.354, 30.9145)
extrude "Extrude53" add 1 faces at (-0.1573, 6.8139, 5.8974) along direction (0, 0, -1) blind 1 on bodies 4 bodies 2 5 6 7 8 4
extrude "Extrude54" add 1 faces at (-5.7275, 6.8139, 1.6983) along direction (0.965926, 0, -0.258819) blind 1 on bodies 5 bodies 2 6 7 8 5
extrude "Extrude55" add 1 faces at (5.4593, 6.8139, 2.5148) along direction (-0.978148, 0, -0.207912) blind 1 on bodies 6 bodies 2 7 8 6
extrude "Extrude56" add 1 faces at (3.6075, 6.8139, -4.8521) along direction (-0.669131, 0, 0.743145) blind 1.5 on bodies 7 bodies 2 8 7
extrude "Extrude57" add 1 faces at (-3.7657, 6.8139, -4.6339) along direction (0.642788, 0, 0.766044) blind 1 on bodies 8 bodies 2 8
